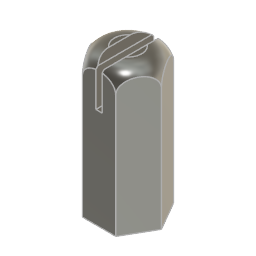
Embroidery Floss Winding Tool for Cordless Screwdriver (Autodesk Fusion 360 design; units mm, degrees)
Autodesk Fusion 360 part; units mm, degrees
sketch "Sketch1" plane through (0, 0, 0) normal (0, 0, 1) x (1, 0, 0)
  line L0 (-1.9341, 3.35) -> (-3.8682, 0)
  line L1 (-3.8682, 0) -> (-1.9341, -3.35)
  line L2 (-1.9341, -3.35) -> (1.9341, -3.35)
  line L3 (1.9341, -3.35) -> (3.8682, 0)
  line L4 (3.8682, 0) -> (1.9341, 3.35)
  line L5 (1.9341, 3.35) -> (-1.9341, 3.35)
  line L6 (-0.6, 5.5) -> (-0.6, -5.5)
  line L7 (0, 2.5) -> (0, 20) construction
  line L8 (0.6, 5.5) -> (0.6, -5.5)
  line L9 (-6.3509, 0) -> (-3.1754, -5.5)
  line L10 (-3.1754, -5.5) -> (3.1754, -5.5)
  line L11 (3.1754, -5.5) -> (6.3509, 0)
  line L12 (6.3509, 0) -> (3.1754, 5.5)
  line L13 (3.1754, 5.5) -> (-3.1754, 5.5)
  line L14 (-3.1754, 5.5) -> (-6.3509, 0)
  dimension "d1" = 6.7
  dimension "d3" = 1.2
  dimension "d14" = 11
  constraint horizontal L5
  constraint perpendicular L5 L6
  constraint symmetric L6.start L7 L8.start
  constraint symmetric L6.end L7 L8.end
  constraint horizontal L13
  constraint coincident L6.start L13
  constraint coincident L6.end L10
  measures "d1" distance of L2 L5
  measures "d3" distance of L6 L8
  measures "d14" distance of L10 L13
extrude "Extrude1" add sketch "Sketch1" along normal blind 13 contours L0 L1 L2 L5 L6 L9 L10 L13 L14 | L5 L6 L8 L13 | L2 L3 L4 L5 L8 L10 L11 L12 L13 | L2 L6 L8 L10
extrude "Extrude2" add sketch "Sketch1" along normal blind 6 from surface at 13
extrude "Extrude3" add sketch "Sketch1" along normal blind 8 from surface at 19 contours L0 L1 L2 L5 L6 | L0 L1 L2 L5 L6 L9 L10 L13 L14 | L2 L3 L4 L5 L8 L10 L11 L12 L13 | L2 L3 L4 L5 L8
chamfer "Chamfer1" distance 1 angle 45 2 edges at (0.6, 0, 27) (-0.6, 0, 27)
sketch "Sketch2" plane through (0, 0, 0) normal (0, 1, 0) x (1, 0, 0)
  line L0 (3.8682, -13) -> (-3.8682, -13)
  line L1 (-3.8682, -13) -> (-3.8682, 0)
  line L2 (-3.8682, 0) -> (-6.3509, 0)
  line L3 (-6.3509, 0) -> (-6.3509, -27)
  line L4 (-6.3509, -27) -> (-1.6, -27)
  line L5 (-1.6, -27) -> (-0.6, -26)
  line L6 (-0.6, -26) -> (-0.6, -19)
  line L7 (-0.6, -19) -> (0.6, -19)
  line L8 (0.6, -19) -> (0.6, -26)
  line L9 (0.6, -26) -> (1.6, -27)
  line L10 (1.6, -27) -> (6.3509, -27)
  line L11 (6.3509, -27) -> (6.3509, 0)
  line L12 (6.3509, 0) -> (3.8682, 0)
  line L13 (3.8682, 0) -> (3.8682, -13)
  line L14 (-1.6, -27) -> (1.6, -27) construction
  line L15 (0, -27) -> (0, -26.8393) construction
  arc A0 (2.6, -27) -> (6.3509, -23.2491) centre (2.6, -23.2491) ccw
  line L16 (3.1754, -27) -> (1.6, -27)
  dimension "d15" = 1
  constraint coincident L4.end L5.start
  constraint coincident L9.end L10.start
  constraint midpoint L14 L15.start
  constraint perpendicular L14 L15
  constraint tangent L11 A0
  constraint coincident L11 A0.end
  constraint coincident L10 A0.start
  constraint tangent A0 L16
  measures "d15" distance of L9.end A0.start
revolve "Revolve1" cut sketch "Sketch2" angle 360 about axis through (0, 0, 1.75) along (0, 0, 1) contours L10 L11 A0 L16
named bodies: "Embroidery Floss Winding Tool for Cordless Screwdriver"
